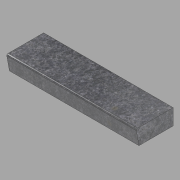
# Autodesk Inventor part: D
Saved by Autodesk Inventor 2022.1 (Build 261234020, 234B)
## iProperties
Created: 2021-12-14
Part Number: D
Material: Granite, Cut, Polished
Document SubType Name: Modeling
Designer: awelt
Density: 2.7 g/cm^3
Appearance: Kasota SN sapphire
Mass: 176785 g
Surface Area: 13386.8 cm^2
Volume: 65476.1 cm^3
Author: awelt
Autodesk Inventor part; units mm, degrees
ref_plane "YZ Plane" through (0, 0, 0) normal (1, 0, 0) x (0, 1, 0)
ref_plane "XZ Plane" through (0, 0, 0) normal (0, 1, 0) x (-1, 0, 0)
ref_plane "XY Plane" through (0, 0, 0) normal (0, 0, 1) x (1, 0, 0)
sketch "Sketch1" plane through (0, 0, 0) normal (1, 0, 0) x (0, 1, 0)
  line L0 (0, 0) -> (0, 152.4)
  line L1 (0, 0) -> (330.2, 0)
  line L2 (0, 152.4) -> (342.9, 152.4)
  line L3 (342.9, 152.4) -> (342.9, 139.7) construction
  arc A0 (355.3918, 137.4098) -> (342.9, 152.4) centre (342.9, 139.7) ccw
  line L4 (330.2, 0) -> (355.7981, 139.6261)
  dimension "d0" = 152.4
  dimension "d1" = 330.2
  dimension "d2" = 342.9
  dimension "d3" = 12.7
  constraints: 10 end point, 2 horizontal, 2 point on circle, 1 centre point, 1 coincident, 1 perpendicular, 1 point on line, 1 tangent, 1 vertical
  measures "d0" distance of L0.start L0.end
  measures "d1" distance of L0.start L1.end
  measures "d2" distance of L0.end L2.end
  measures "d3" distance of L2.end L3.end
extrude "Extrusion1" add sketch "Sketch1" along normal blind 1249.5609
body "Solid1"
